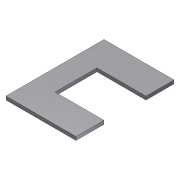
# Autodesk Inventor part: PitchingArmConcept
Saved by Autodesk Inventor 2012 (Build 160160000, 160)
## iProperties
Created: 2012-01-19
Part Number: PitchingArmConcept
Material: Default
Document SubType Name: Modeling
Designer: JesseK
Density: 1 g/cm^3
Mass: 100.213 g
Surface Area: 366.143 cm^2
Volume: 100.213 cm^3
Author: JesseK
Autodesk Inventor part; units mm, degrees
ref_plane "YZ Plane" through (0, 0, 0) normal (1, 0, 0) x (0, 1, 0)
ref_plane "XZ Plane" through (0, 0, 0) normal (0, 1, 0) x (-1, 0, 0)
ref_plane "XY Plane" through (0, 0, 0) normal (0, 0, 1) x (1, 0, 0)
sketch "Sketch1" plane through (0, 0, 0) normal (0, 0, 1) x (1, 0, 0)
  arc A0 (23.9202, -3.175) -> (23.9202, 3.175) centre (0, 0) ccw
  line L0 (23.9202, 3.175) -> (150.9202, 3.175)
  line L1 (150.9202, 3.175) -> (150.9202, -3.175)
  line L2 (150.9202, -3.175) -> (23.9202, -3.175)
  line L3 (23.9202, 3.175) -> (0, 3.175) construction
  line L4 (0, 0) -> (0, 3.175) construction
  line L5 (0, 0) -> (0, -3.175) construction
  line L6 (0, -3.175) -> (23.9202, -3.175) construction
  dimension "d0" = 24.13
  dimension "d1" = 6.35
  dimension "d9" = 127
  constraints: 14 end point, 4 horizontal, 3 vertical, 2 point on circle, 1 centre point, 1 coincident, 1 collinear
  measures "d0" radius of A0
  measures "d1" distance of L0.end L1.end
  measures "d9" distance of L0.start L0.end
extrude "Extrusion1" add sketch "Sketch1" along normal blind 177.8
sketch "Sketch2" plane through (23.9202, 3.175, 0) normal (0, 1, 0) x (1, 0, 0)
  line L0 (0, -177.8) -> (127, -177.8) projected
  line L1 (127, 0) -> (127, -177.8) projected
  line L2 (0, 0) -> (127, 0) projected
  line L3 (127, -50.8) -> (38.1, -50.8)
  line L4 (38.1, -50.8) -> (38.1, -127)
  line L5 (38.1, -127) -> (127, -127)
  line L6 (127, -127) -> (127, -50.8)
  line L7 (38.1, -50.8) -> (38.1, 0) construction
  line L8 (38.1, -127) -> (38.1, -177.8) construction
  line L9 (0, 0) -> (0, -177.8) projected
  point P0 (-23.9202, 0)
  dimension "d4" = 76.2
  dimension "d8" = 38.1
  constraints: 12 end point, 3 point on line, 2 parallel, 2 vertical, 1 collinear, 1 horizontal, 1 perpendicular
  measures "d4" distance of L3.end L4.end
  measures "d8" distance between parallel lines of L9 L4
extrude "Extrusion2" cut sketch "Sketch2" against normal up to next contours L5 L4 L3 L1
body "Solid1"
